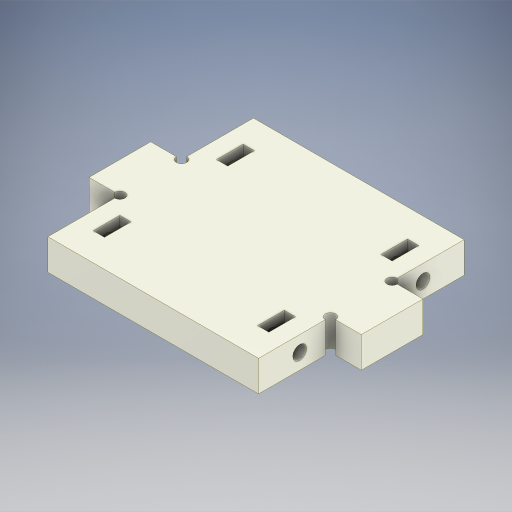
# Autodesk Inventor part: hand connection
Saved by Autodesk Inventor 2024 (Build 280153000, 153)
## iProperties
Created: 2024-09-04
Part Number: hand connection
Material: PMMA 플라스틱
Document SubType Name: Modeling
Designer: msi
Density: 1.188 g/cm^3
Appearance: 매끄러움 - 아이보리색
Author: msi
Autodesk Inventor part; units mm, degrees
ref_plane "우측면도" through (0, 0, 0) normal (1, 0, 0) x (0, 1, 0)
ref_plane "평면도" through (0, 0, 0) normal (0, 1, 0) x (-1, 0, 0)
ref_plane "정면도" through (0, 0, 0) normal (0, 0, 1) x (1, 0, 0)
sketch "스케치1" plane through (0, 0, 0) normal (0, 1, 0) x (-1, 0, 0)
  line L0 (-20.5, 15) -> (20.5, 15)
  line L1 (20.5, 15) -> (20.5, -15)
  line L2 (20.5, -15) -> (-20.5, -15)
  line L3 (-20.5, -15) -> (-20.5, 15)
  line L4 (-20.5, 15) -> (20.5, -15) construction
  line L5 (20.5, 15) -> (-20.5, -15) construction
  line L6 (9, -15) -> (-9, -15)
  line L7 (9, 15) -> (-9, 15)
  line L8 (20.5, -3) -> (20.5, 15)
  line L9 (-20.5, -3) -> (-20.5, 15)
  line L10 (20.5, 6) -> (26.5, 6)
  line L11 (26.5, 6) -> (26.5, -6)
  line L12 (26.5, -6) -> (20.5, -6)
  line L13 (20.5, -6) -> (20.5, 6)
  line L14 (-20.5, 6) -> (-26.5, 6)
  line L15 (-26.5, 6) -> (-26.5, -6)
  line L16 (-26.5, -6) -> (-20.5, -6)
  line L17 (-20.5, -6) -> (-20.5, 6)
  point P0 (0, 0)
  dimension "d0" = 41
  dimension "d1" = 30
  dimension "d16" = 6
  dimension "d17" = 12
  dimension "d18" = 6
  dimension "d19" = 12
  constraints: 36 end point, 6 parallel, 5 horizontal, 4 midpoint, 4 point on line, 3 perpendicular
  measures "d0" distance of L1.end L2.end
  measures "d1" distance of L0.end L1.end
  measures "d16" distance of L11.end L12.end
  measures "d17" distance of L10.end L11.end
  measures "d18" distance of L16.end L15.end
  measures "d19" distance of L15.end L14.end
extrude "돌출3" add sketch "스케치1" along normal blind 6
sketch "스케치3" plane through (26.5, 0, 6) normal (1, 0, 0) x (0, 0, -1)
  circle A0 centre (18, 3) radius 1.35
  circle A1 centre (-6, 3) radius 1.35
  point P0 (6, 0)
  dimension "d22" = 2.7
  dimension "d23" = 2.7
  constraints: 2 centre point
  measures "d22" diameter of A0
  measures "d23" diameter of A1
extrude "돌출4" cut sketch "스케치3" against normal blind 100
sketch "스케치4" plane through (0, 6, 0) normal (0, 1, 0) x (1, 0, 0)
  line L0 (20.5, -10.65) -> (-20.5, -10.65) projected
  line L1 (20.5, -13.35) -> (-20.5, -13.35) projected
  line L2 (20.5, 10.65) -> (-20.5, 10.65) projected
  line L3 (20.5, 13.35) -> (-20.5, 13.35) projected
  line L4 (16, -13.35) -> (42.7, -13.35) construction
  line L5 (16, -13.35) -> (16, -10.65)
  line L6 (16, 10.65) -> (16, 13.35)
  line L7 (17.1, -14.6) -> (14.9, -14.6)
  line L8 (14.9, -14.6) -> (14.9, -9.4)
  line L9 (14.9, -9.4) -> (17.1, -9.4)
  line L10 (17.1, -9.4) -> (17.1, -14.6)
  line L11 (17.1, -14.6) -> (14.9, -9.4) construction
  line L12 (14.9, -14.6) -> (17.1, -9.4) construction
  line L13 (-17.1, -14.6) -> (-14.9, -14.6)
  line L14 (-14.9, -14.6) -> (-14.9, -9.4)
  line L15 (-14.9, -9.4) -> (-17.1, -9.4)
  line L16 (-17.1, -9.4) -> (-17.1, -14.6)
  line L17 (-17.1, -14.6) -> (-14.9, -9.4) construction
  line L18 (-14.9, -14.6) -> (-17.1, -9.4) construction
  line L19 (-14.9, 14.6) -> (-17.1, 14.6)
  line L20 (-17.1, 14.6) -> (-17.1, 9.4)
  line L21 (-17.1, 9.4) -> (-14.9, 9.4)
  line L22 (-14.9, 9.4) -> (-14.9, 14.6)
  line L23 (-14.9, 14.6) -> (-17.1, 9.4) construction
  line L24 (-17.1, 14.6) -> (-14.9, 9.4) construction
  line L25 (17.1, 9.4) -> (14.9, 9.4)
  line L26 (14.9, 9.4) -> (14.9, 14.6)
  line L27 (14.9, 14.6) -> (17.1, 14.6)
  line L28 (17.1, 14.6) -> (17.1, 9.4)
  line L29 (17.1, 9.4) -> (14.9, 14.6) construction
  line L30 (14.9, 9.4) -> (17.1, 14.6) construction
  point P0 (0, 0)
  point P1 (16, -12)
  point P2 (-16, -12)
  point P3 (-16, 12)
  point P4 (16, 12)
  dimension "d39" = 5
  dimension "d27" = 2.2
  dimension "d28" = 5.2
  dimension "d29" = 2.2
  dimension "d30" = 5.2
  dimension "d31" = 2.2
  dimension "d32" = 5.2
  dimension "d33" = 2.2
  dimension "d34" = 5.2
  constraints: 54 end point, 9 midpoint, 8 parallel, 5 horizontal, 4 perpendicular, 4 point on line
  measures "d27" distance of L8.end L9.end
  measures "d28" distance of L7.end L8.end
  measures "d29" distance of L15.end L14.end
  measures "d30" distance of L14.end L13.end
  measures "d31" distance of L21.end L20.end
  measures "d32" distance of L20.end L19.end
  measures "d33" distance of L26.end L27.end
  measures "d34" distance of L25.end L26.end
extrude "돌출5" cut sketch "스케치4" against normal blind 100 contours L10 L1 L5 L0 | L0 L8 L9 L10 | L5 L1 L8 L0 | L10 L7 L8 L1 | L14 L1 L16 L0 | L0 L16 L15 L14 | L14 L13 L16 L1 | L28 L25 L26 L2 | L2 L6 L3 L28 | L2 L26 L3 L6 | L3 L26 L27 L28 | L22 L21 L20 L2 | L2 L20 L3 L22 | L3 L20 L19 L22
sketch "스케치5" plane through (20.5, 0, -15) normal (0, 0, -1) x (-1, 0, 0)
  line L0 (0, 0) -> (41, 0)
  line L1 (41, 0) -> (41, 6)
  line L2 (41, 6) -> (0, 6)
  line L3 (0, 6) -> (0, 0)
  point P0 (20.5, 0)
  dimension "d37" = 41
  dimension "d38" = 6
  constraints: 8 end point, 2 parallel, 1 horizontal, 1 perpendicular
  measures "d37" distance of L2.end L1.end
  measures "d38" distance of L1.end L0.end
extrude "돌출6" add sketch "스케치5" along normal blind 5
sketch "스케치6" plane through (-20.5, 0, 15) normal (0, 0, 1) x (1, 0, 0)
  line L0 (0, 0) -> (41, 0)
  line L1 (41, 0) -> (41, 6)
  line L2 (41, 6) -> (0, 6)
  line L3 (0, 6) -> (0, 0)
  point P0 (20.5, 0)
  dimension "d41" = 41
  dimension "d42" = 6
  constraints: 8 end point, 2 parallel, 1 horizontal, 1 perpendicular
  measures "d41" distance of L2.end L1.end
  measures "d42" distance of L1.end L0.end
extrude "돌출7" add sketch "스케치6" along normal blind 5
sketch "스케치7" plane through (0, 6, 0) normal (0, 1, 0) x (1, 0, 0)
  line L0 (17.1, 14.6) -> (17.1, 9.4) projected
  line L1 (17.1, 9.4) -> (14.9, 9.4) projected
  line L2 (14.9, 9.4) -> (14.9, 14.6) projected
  line L3 (14.9, 14.6) -> (17.1, 14.6) projected
  line L4 (-14.9, -9.4) -> (-14.9, -14.6) projected
  line L5 (-14.9, -14.6) -> (-17.1, -14.6) projected
  line L6 (-17.1, -14.6) -> (-17.1, -9.4) projected
  line L7 (-17.1, -9.4) -> (-14.9, -9.4) projected
  line L8 (-17.1, 14.6) -> (-14.9, 14.6) projected
  line L9 (-14.9, 14.6) -> (-14.9, 9.4) projected
  line L10 (-14.9, 9.4) -> (-17.1, 9.4) projected
  line L11 (-17.1, 9.4) -> (-17.1, 14.6) projected
  line L12 (17.1, -9.4) -> (17.1, -14.6) projected
  line L13 (17.1, -14.6) -> (14.9, -14.6) projected
  line L14 (14.9, -14.6) -> (14.9, -9.4) projected
  line L15 (14.9, -9.4) -> (17.1, -9.4) projected
  line L16 (-20.5, 6) -> (-20.5, 20) projected
  line L17 (-20.5, 6) -> (-26.5, 6) projected
  line L18 (-26.5, 6) -> (-26.5, -6) projected
  line L19 (-26.5, -6) -> (-20.5, -6) projected
  line L20 (-20.5, -6) -> (-20.5, -20) projected
  line L21 (20.5, -20) -> (-20.5, -20) projected
  line L22 (20.5, -6) -> (20.5, -20) projected
  line L23 (20.5, -6) -> (26.5, -6) projected
  line L24 (26.5, -6) -> (26.5, 6) projected
  line L25 (26.5, 6) -> (20.5, 6) projected
  line L26 (20.5, 6) -> (20.5, 20) projected
  line L27 (-20.5, 20) -> (20.5, 20) projected
  circle A0 centre (-20.5, 6) radius 1
  circle A1 centre (-20.5, -6) radius 1
  circle A2 centre (20.5, 6) radius 1
  circle A3 centre (20.5, -6) radius 1
  point P0 (0, 0)
  point P1 (-21.5, -6)
  point P2 (-20.5, -7)
  point P3 (20.5, -7)
  point P4 (21.5, -6)
  point P5 (21.5, 6)
  point P6 (20.5, 7)
  point P7 (-20.5, 7)
  point P8 (-21.5, 6)
  dimension "d45" = 2
  dimension "d46" = 2
  dimension "d47" = 2
  dimension "d48" = 2
  constraints: 4 centre point, 4 coincident
  measures "d45" diameter of A0
  measures "d46" diameter of A1
  measures "d47" diameter of A2
  measures "d48" diameter of A3
extrude "돌출9" cut sketch "스케치7" against normal blind 10 contours L17 A0 L16 | L16 A0 L17 | A2 L25 L26 | L26 L25 A2 | A1 L20 L19 | L19 L20 A1 | A3 L22 L23 | L23 L22 A3
